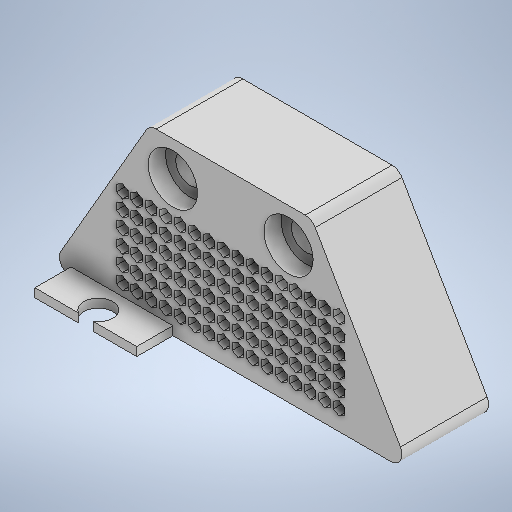
# Autodesk Inventor part: EngineMount
Saved by Autodesk Inventor 2026.1 (Build 301233020, 233B)
## iProperties
Created: 2025-10-14
Part Number: EngineMount
Material: Generic
Document SubType Name: Modeling
Designer: yo
Density: 1 g/cm^3
Appearance: Default
Author: yo
Autodesk Inventor part; units mm, degrees
ref_plane "YZ Plane" through (0, 0, 0) normal (1, 0, 0) x (0, 1, 0)
ref_plane "XZ Plane" through (0, 0, 0) normal (0, 1, 0) x (-1, 0, 0)
ref_plane "XY Plane" through (0, 0, 0) normal (0, 0, 1) x (1, 0, 0)
sketch "Sketch1" plane through (0, 0, 0) normal (0, 0, 1) x (1, 0, 0)
  line L0 (-55.2184, 0) -> (55.2184, 0)
  line L1 (-25.7735, 59) -> (25.7735, 59)
  circle A0 centre (-20, 47) radius 8.5
  line L2 (0, 59) -> (0, 0) construction
  circle A1 centre (-20, 47) radius 5
  circle A2 centre (20, 47) radius 8.5
  circle A3 centre (20, 47) radius 5
  arc A4 (-58.6825, 6) -> (-55.2184, 0) centre (-55.2184, 4) ccw
  arc A5 (-25.7735, 59) -> (-29.2376, 57) centre (-25.7735, 55) ccw
  line L3 (-58.6825, 6) -> (-29.2376, 57)
  arc A6 (55.2184, 0) -> (58.6825, 6) centre (55.2184, 4) ccw
  arc A7 (29.2376, 57) -> (25.7735, 59) centre (25.7735, 55) ccw
  line L4 (58.6825, 6) -> (29.2376, 57)
  line L5 (-55.2184, 3) -> (-20, 3)
  line L6 (-20, 3) -> (-20, 0)
  line L7 (-20, 0) -> (-55.2184, 0)
  line L8 (-55.2184, 0) -> (-55.2184, 3)
  line L9 (-35.5, 33.3453) -> (-37.5, 32.1906)
  line L10 (-37.5, 32.1906) -> (-39.5, 33.3453)
  line L11 (-39.5, 33.3453) -> (-39.5, 35.6547)
  line L12 (-39.5, 35.6547) -> (-37.5, 36.8094)
  line L13 (-37.5, 36.8094) -> (-35.5, 35.6547)
  line L14 (-35.5, 35.6547) -> (-35.5, 33.3453)
  line L15 (-32.5, 36.8094) -> (-30.5, 35.6547)
  line L16 (-34.5, 33.3453) -> (-34.5, 35.6547)
  line L17 (-30.5, 35.6547) -> (-30.5, 33.3453)
  line L18 (-32.5, 32.1906) -> (-34.5, 33.3453)
  line L19 (-30.5, 33.3453) -> (-32.5, 32.1906)
  line L20 (-34.5, 35.6547) -> (-32.5, 36.8094)
  line L21 (-27.5, 36.8094) -> (-25.5, 35.6547)
  line L22 (-29.5, 33.3453) -> (-29.5, 35.6547)
  line L23 (-25.5, 35.6547) -> (-25.5, 33.3453)
  line L24 (-27.5, 32.1906) -> (-29.5, 33.3453)
  line L25 (-25.5, 33.3453) -> (-27.5, 32.1906)
  line L26 (-29.5, 35.6547) -> (-27.5, 36.8094)
  line L27 (-22.5, 36.8094) -> (-20.5, 35.6547)
  line L28 (-24.5, 33.3453) -> (-24.5, 35.6547)
  line L29 (-20.5, 35.6547) -> (-20.5, 33.3453)
  line L30 (-22.5, 32.1906) -> (-24.5, 33.3453)
  line L31 (-20.5, 33.3453) -> (-22.5, 32.1906)
  line L32 (-24.5, 35.6547) -> (-22.5, 36.8094)
  line L33 (-17.5, 36.8094) -> (-15.5, 35.6547)
  line L34 (-19.5, 33.3453) -> (-19.5, 35.6547)
  line L35 (-15.5, 35.6547) -> (-15.5, 33.3453)
  line L36 (-17.5, 32.1906) -> (-19.5, 33.3453)
  line L37 (-15.5, 33.3453) -> (-17.5, 32.1906)
  line L38 (-19.5, 35.6547) -> (-17.5, 36.8094)
  line L39 (-12.5, 36.8094) -> (-10.5, 35.6547)
  line L40 (-14.5, 33.3453) -> (-14.5, 35.6547)
  line L41 (-10.5, 35.6547) -> (-10.5, 33.3453)
  line L42 (-12.5, 32.1906) -> (-14.5, 33.3453)
  line L43 (-10.5, 33.3453) -> (-12.5, 32.1906)
  line L44 (-14.5, 35.6547) -> (-12.5, 36.8094)
  line L45 (-7.5, 36.8094) -> (-5.5, 35.6547)
  line L46 (-9.5, 33.3453) -> (-9.5, 35.6547)
  line L47 (-5.5, 35.6547) -> (-5.5, 33.3453)
  line L48 (-7.5, 32.1906) -> (-9.5, 33.3453)
  line L49 (-5.5, 33.3453) -> (-7.5, 32.1906)
  line L50 (-9.5, 35.6547) -> (-7.5, 36.8094)
  line L51 (-2.5, 36.8094) -> (-0.5, 35.6547)
  line L52 (-4.5, 33.3453) -> (-4.5, 35.6547)
  line L53 (-0.5, 35.6547) -> (-0.5, 33.3453)
  line L54 (-2.5, 32.1906) -> (-4.5, 33.3453)
  line L55 (-0.5, 33.3453) -> (-2.5, 32.1906)
  line L56 (-4.5, 35.6547) -> (-2.5, 36.8094)
  line L57 (2.5, 36.8094) -> (4.5, 35.6547)
  line L58 (0.5, 33.3453) -> (0.5, 35.6547)
  line L59 (4.5, 35.6547) -> (4.5, 33.3453)
  line L60 (2.5, 32.1906) -> (0.5, 33.3453)
  line L61 (4.5, 33.3453) -> (2.5, 32.1906)
  line L62 (0.5, 35.6547) -> (2.5, 36.8094)
  line L63 (7.5, 36.8094) -> (9.5, 35.6547)
  line L64 (5.5, 33.3453) -> (5.5, 35.6547)
  line L65 (9.5, 35.6547) -> (9.5, 33.3453)
  line L66 (7.5, 32.1906) -> (5.5, 33.3453)
  line L67 (9.5, 33.3453) -> (7.5, 32.1906)
  line L68 (5.5, 35.6547) -> (7.5, 36.8094)
  line L69 (12.5, 36.8094) -> (14.5, 35.6547)
  line L70 (10.5, 33.3453) -> (10.5, 35.6547)
  line L71 (14.5, 35.6547) -> (14.5, 33.3453)
  line L72 (12.5, 32.1906) -> (10.5, 33.3453)
  line L73 (14.5, 33.3453) -> (12.5, 32.1906)
  line L74 (10.5, 35.6547) -> (12.5, 36.8094)
  line L75 (17.5, 36.8094) -> (19.5, 35.6547)
  line L76 (15.5, 33.3453) -> (15.5, 35.6547)
  line L77 (19.5, 35.6547) -> (19.5, 33.3453)
  line L78 (17.5, 32.1906) -> (15.5, 33.3453)
  line L79 (19.5, 33.3453) -> (17.5, 32.1906)
  line L80 (15.5, 35.6547) -> (17.5, 36.8094)
  line L81 (22.5, 36.8094) -> (24.5, 35.6547)
  line L82 (20.5, 33.3453) -> (20.5, 35.6547)
  line L83 (24.5, 35.6547) -> (24.5, 33.3453)
  line L84 (22.5, 32.1906) -> (20.5, 33.3453)
  line L85 (24.5, 33.3453) -> (22.5, 32.1906)
  line L86 (20.5, 35.6547) -> (22.5, 36.8094)
  line L87 (27.5, 36.8094) -> (29.5, 35.6547)
  line L88 (25.5, 33.3453) -> (25.5, 35.6547)
  line L89 (29.5, 35.6547) -> (29.5, 33.3453)
  line L90 (27.5, 32.1906) -> (25.5, 33.3453)
  line L91 (29.5, 33.3453) -> (27.5, 32.1906)
  line L92 (25.5, 35.6547) -> (27.5, 36.8094)
  line L93 (32.5, 36.8094) -> (34.5, 35.6547)
  line L94 (30.5, 33.3453) -> (30.5, 35.6547)
  line L95 (34.5, 35.6547) -> (34.5, 33.3453)
  line L96 (32.5, 32.1906) -> (30.5, 33.3453)
  line L97 (34.5, 33.3453) -> (32.5, 32.1906)
  line L98 (30.5, 35.6547) -> (32.5, 36.8094)
  line L99 (37.5, 36.8094) -> (39.5, 35.6547)
  line L100 (35.5, 33.3453) -> (35.5, 35.6547)
  line L101 (39.5, 35.6547) -> (39.5, 33.3453)
  line L102 (37.5, 32.1906) -> (35.5, 33.3453)
  line L103 (39.5, 33.3453) -> (37.5, 32.1906)
  line L104 (35.5, 35.6547) -> (37.5, 36.8094)
  line L105 (-37.5, 31.3094) -> (-35.5, 30.1547)
  line L106 (-39.5, 27.8453) -> (-39.5, 30.1547)
  line L107 (-35.5, 30.1547) -> (-35.5, 27.8453)
  line L108 (-37.5, 26.6906) -> (-39.5, 27.8453)
  line L109 (-35.5, 27.8453) -> (-37.5, 26.6906)
  line L110 (-39.5, 30.1547) -> (-37.5, 31.3094)
  line L111 (-32.5, 31.3094) -> (-30.5, 30.1547)
  line L112 (-34.5, 27.8453) -> (-34.5, 30.1547)
  line L113 (-30.5, 30.1547) -> (-30.5, 27.8453)
  line L114 (-32.5, 26.6906) -> (-34.5, 27.8453)
  line L115 (-30.5, 27.8453) -> (-32.5, 26.6906)
  line L116 (-34.5, 30.1547) -> (-32.5, 31.3094)
  line L117 (-27.5, 31.3094) -> (-25.5, 30.1547)
  line L118 (-29.5, 27.8453) -> (-29.5, 30.1547)
  line L119 (-25.5, 30.1547) -> (-25.5, 27.8453)
  line L120 (-27.5, 26.6906) -> (-29.5, 27.8453)
  line L121 (-25.5, 27.8453) -> (-27.5, 26.6906)
  line L122 (-29.5, 30.1547) -> (-27.5, 31.3094)
  line L123 (-22.5, 31.3094) -> (-20.5, 30.1547)
  line L124 (-24.5, 27.8453) -> (-24.5, 30.1547)
  line L125 (-20.5, 30.1547) -> (-20.5, 27.8453)
  line L126 (-22.5, 26.6906) -> (-24.5, 27.8453)
  line L127 (-20.5, 27.8453) -> (-22.5, 26.6906)
  line L128 (-24.5, 30.1547) -> (-22.5, 31.3094)
  line L129 (-17.5, 31.3094) -> (-15.5, 30.1547)
  line L130 (-19.5, 27.8453) -> (-19.5, 30.1547)
  line L131 (-15.5, 30.1547) -> (-15.5, 27.8453)
  line L132 (-17.5, 26.6906) -> (-19.5, 27.8453)
  line L133 (-15.5, 27.8453) -> (-17.5, 26.6906)
  line L134 (-19.5, 30.1547) -> (-17.5, 31.3094)
  line L135 (-12.5, 31.3094) -> (-10.5, 30.1547)
  line L136 (-14.5, 27.8453) -> (-14.5, 30.1547)
  line L137 (-10.5, 30.1547) -> (-10.5, 27.8453)
  line L138 (-12.5, 26.6906) -> (-14.5, 27.8453)
  line L139 (-10.5, 27.8453) -> (-12.5, 26.6906)
  line L140 (-14.5, 30.1547) -> (-12.5, 31.3094)
  line L141 (-7.5, 31.3094) -> (-5.5, 30.1547)
  line L142 (-9.5, 27.8453) -> (-9.5, 30.1547)
  line L143 (-5.5, 30.1547) -> (-5.5, 27.8453)
  line L144 (-7.5, 26.6906) -> (-9.5, 27.8453)
  line L145 (-5.5, 27.8453) -> (-7.5, 26.6906)
  line L146 (-9.5, 30.1547) -> (-7.5, 31.3094)
  line L147 (-2.5, 31.3094) -> (-0.5, 30.1547)
  line L148 (-4.5, 27.8453) -> (-4.5, 30.1547)
  line L149 (-0.5, 30.1547) -> (-0.5, 27.8453)
  line L150 (-2.5, 26.6906) -> (-4.5, 27.8453)
  line L151 (-0.5, 27.8453) -> (-2.5, 26.6906)
  line L152 (-4.5, 30.1547) -> (-2.5, 31.3094)
  line L153 (2.5, 31.3094) -> (4.5, 30.1547)
  line L154 (0.5, 27.8453) -> (0.5, 30.1547)
  line L155 (4.5, 30.1547) -> (4.5, 27.8453)
  line L156 (2.5, 26.6906) -> (0.5, 27.8453)
  line L157 (4.5, 27.8453) -> (2.5, 26.6906)
  line L158 (0.5, 30.1547) -> (2.5, 31.3094)
  line L159 (7.5, 31.3094) -> (9.5, 30.1547)
  line L160 (5.5, 27.8453) -> (5.5, 30.1547)
  line L161 (9.5, 30.1547) -> (9.5, 27.8453)
  line L162 (7.5, 26.6906) -> (5.5, 27.8453)
  line L163 (9.5, 27.8453) -> (7.5, 26.6906)
  line L164 (5.5, 30.1547) -> (7.5, 31.3094)
  line L165 (12.5, 31.3094) -> (14.5, 30.1547)
  line L166 (10.5, 27.8453) -> (10.5, 30.1547)
  line L167 (14.5, 30.1547) -> (14.5, 27.8453)
  line L168 (12.5, 26.6906) -> (10.5, 27.8453)
  line L169 (14.5, 27.8453) -> (12.5, 26.6906)
  line L170 (10.5, 30.1547) -> (12.5, 31.3094)
  line L171 (17.5, 31.3094) -> (19.5, 30.1547)
  line L172 (15.5, 27.8453) -> (15.5, 30.1547)
  line L173 (19.5, 30.1547) -> (19.5, 27.8453)
  line L174 (17.5, 26.6906) -> (15.5, 27.8453)
  line L175 (19.5, 27.8453) -> (17.5, 26.6906)
  line L176 (15.5, 30.1547) -> (17.5, 31.3094)
  line L177 (22.5, 31.3094) -> (24.5, 30.1547)
  line L178 (20.5, 27.8453) -> (20.5, 30.1547)
  line L179 (24.5, 30.1547) -> (24.5, 27.8453)
  line L180 (22.5, 26.6906) -> (20.5, 27.8453)
  line L181 (24.5, 27.8453) -> (22.5, 26.6906)
  line L182 (20.5, 30.1547) -> (22.5, 31.3094)
  line L183 (27.5, 31.3094) -> (29.5, 30.1547)
  line L184 (25.5, 27.8453) -> (25.5, 30.1547)
  line L185 (29.5, 30.1547) -> (29.5, 27.8453)
  line L186 (27.5, 26.6906) -> (25.5, 27.8453)
  line L187 (29.5, 27.8453) -> (27.5, 26.6906)
  line L188 (25.5, 30.1547) -> (27.5, 31.3094)
  line L189 (32.5, 31.3094) -> (34.5, 30.1547)
  line L190 (30.5, 27.8453) -> (30.5, 30.1547)
  line L191 (34.5, 30.1547) -> (34.5, 27.8453)
  line L192 (32.5, 26.6906) -> (30.5, 27.8453)
  line L193 (34.5, 27.8453) -> (32.5, 26.6906)
  line L194 (30.5, 30.1547) -> (32.5, 31.3094)
  line L195 (37.5, 31.3094) -> (39.5, 30.1547)
  line L196 (35.5, 27.8453) -> (35.5, 30.1547)
  line L197 (39.5, 30.1547) -> (39.5, 27.8453)
  line L198 (37.5, 26.6906) -> (35.5, 27.8453)
  line L199 (39.5, 27.8453) -> (37.5, 26.6906)
  line L200 (35.5, 30.1547) -> (37.5, 31.3094)
  line L201 (-37.5, 25.8094) -> (-35.5, 24.6547)
  line L202 (-39.5, 22.3453) -> (-39.5, 24.6547)
  line L203 (-35.5, 24.6547) -> (-35.5, 22.3453)
  line L204 (-37.5, 21.1906) -> (-39.5, 22.3453)
  line L205 (-35.5, 22.3453) -> (-37.5, 21.1906)
  line L206 (-39.5, 24.6547) -> (-37.5, 25.8094)
  line L207 (-32.5, 25.8094) -> (-30.5, 24.6547)
  line L208 (-34.5, 22.3453) -> (-34.5, 24.6547)
  line L209 (-30.5, 24.6547) -> (-30.5, 22.3453)
  line L210 (-32.5, 21.1906) -> (-34.5, 22.3453)
  line L211 (-30.5, 22.3453) -> (-32.5, 21.1906)
  line L212 (-34.5, 24.6547) -> (-32.5, 25.8094)
  line L213 (-27.5, 25.8094) -> (-25.5, 24.6547)
  line L214 (-29.5, 22.3453) -> (-29.5, 24.6547)
  line L215 (-25.5, 24.6547) -> (-25.5, 22.3453)
  line L216 (-27.5, 21.1906) -> (-29.5, 22.3453)
  line L217 (-25.5, 22.3453) -> (-27.5, 21.1906)
  line L218 (-29.5, 24.6547) -> (-27.5, 25.8094)
  line L219 (-22.5, 25.8094) -> (-20.5, 24.6547)
  line L220 (-24.5, 22.3453) -> (-24.5, 24.6547)
  line L221 (-20.5, 24.6547) -> (-20.5, 22.3453)
  line L222 (-22.5, 21.1906) -> (-24.5, 22.3453)
  line L223 (-20.5, 22.3453) -> (-22.5, 21.1906)
  line L224 (-24.5, 24.6547) -> (-22.5, 25.8094)
  line L225 (-17.5, 25.8094) -> (-15.5, 24.6547)
  line L226 (-19.5, 22.3453) -> (-19.5, 24.6547)
  line L227 (-15.5, 24.6547) -> (-15.5, 22.3453)
  line L228 (-17.5, 21.1906) -> (-19.5, 22.3453)
  line L229 (-15.5, 22.3453) -> (-17.5, 21.1906)
  line L230 (-19.5, 24.6547) -> (-17.5, 25.8094)
  line L231 (-12.5, 25.8094) -> (-10.5, 24.6547)
  line L232 (-14.5, 22.3453) -> (-14.5, 24.6547)
  line L233 (-10.5, 24.6547) -> (-10.5, 22.3453)
  line L234 (-12.5, 21.1906) -> (-14.5, 22.3453)
  line L235 (-10.5, 22.3453) -> (-12.5, 21.1906)
  line L236 (-14.5, 24.6547) -> (-12.5, 25.8094)
  line L237 (-7.5, 25.8094) -> (-5.5, 24.6547)
  line L238 (-9.5, 22.3453) -> (-9.5, 24.6547)
  line L239 (-5.5, 24.6547) -> (-5.5, 22.3453)
  line L240 (-7.5, 21.1906) -> (-9.5, 22.3453)
  line L241 (-5.5, 22.3453) -> (-7.5, 21.1906)
  line L242 (-9.5, 24.6547) -> (-7.5, 25.8094)
  line L243 (-2.5, 25.8094) -> (-0.5, 24.6547)
  line L244 (-4.5, 22.3453) -> (-4.5, 24.6547)
  line L245 (-0.5, 24.6547) -> (-0.5, 22.3453)
  line L246 (-2.5, 21.1906) -> (-4.5, 22.3453)
  line L247 (-0.5, 22.3453) -> (-2.5, 21.1906)
  line L248 (-4.5, 24.6547) -> (-2.5, 25.8094)
  line L249 (2.5, 25.8094) -> (4.5, 24.6547)
  line L250 (0.5, 22.3453) -> (0.5, 24.6547)
  line L251 (4.5, 24.6547) -> (4.5, 22.3453)
  line L252 (2.5, 21.1906) -> (0.5, 22.3453)
  line L253 (4.5, 22.3453) -> (2.5, 21.1906)
  line L254 (0.5, 24.6547) -> (2.5, 25.8094)
  line L255 (7.5, 25.8094) -> (9.5, 24.6547)
  line L256 (5.5, 22.3453) -> (5.5, 24.6547)
  line L257 (9.5, 24.6547) -> (9.5, 22.3453)
  line L258 (7.5, 21.1906) -> (5.5, 22.3453)
  line L259 (9.5, 22.3453) -> (7.5, 21.1906)
  line L260 (5.5, 24.6547) -> (7.5, 25.8094)
  line L261 (12.5, 25.8094) -> (14.5, 24.6547)
  line L262 (10.5, 22.3453) -> (10.5, 24.6547)
  line L263 (14.5, 24.6547) -> (14.5, 22.3453)
  line L264 (12.5, 21.1906) -> (10.5, 22.3453)
  line L265 (14.5, 22.3453) -> (12.5, 21.1906)
  line L266 (10.5, 24.6547) -> (12.5, 25.8094)
  line L267 (17.5, 25.8094) -> (19.5, 24.6547)
  line L268 (15.5, 22.3453) -> (15.5, 24.6547)
  line L269 (19.5, 24.6547) -> (19.5, 22.3453)
  line L270 (17.5, 21.1906) -> (15.5, 22.3453)
  line L271 (19.5, 22.3453) -> (17.5, 21.1906)
  line L272 (15.5, 24.6547) -> (17.5, 25.8094)
  line L273 (22.5, 25.8094) -> (24.5, 24.6547)
  line L274 (20.5, 22.3453) -> (20.5, 24.6547)
  line L275 (24.5, 24.6547) -> (24.5, 22.3453)
  line L276 (22.5, 21.1906) -> (20.5, 22.3453)
  line L277 (24.5, 22.3453) -> (22.5, 21.1906)
  line L278 (20.5, 24.6547) -> (22.5, 25.8094)
  line L279 (27.5, 25.8094) -> (29.5, 24.6547)
  line L280 (25.5, 22.3453) -> (25.5, 24.6547)
  line L281 (29.5, 24.6547) -> (29.5, 22.3453)
  line L282 (27.5, 21.1906) -> (25.5, 22.3453)
  line L283 (29.5, 22.3453) -> (27.5, 21.1906)
  line L284 (25.5, 24.6547) -> (27.5, 25.8094)
  line L285 (32.5, 25.8094) -> (34.5, 24.6547)
  line L286 (30.5, 22.3453) -> (30.5, 24.6547)
  line L287 (34.5, 24.6547) -> (34.5, 22.3453)
  line L288 (32.5, 21.1906) -> (30.5, 22.3453)
  line L289 (34.5, 22.3453) -> (32.5, 21.1906)
  line L290 (30.5, 24.6547) -> (32.5, 25.8094)
  line L291 (37.5, 25.8094) -> (39.5, 24.6547)
  line L292 (35.5, 22.3453) -> (35.5, 24.6547)
  line L293 (39.5, 24.6547) -> (39.5, 22.3453)
  line L294 (37.5, 21.1906) -> (35.5, 22.3453)
  line L295 (39.5, 22.3453) -> (37.5, 21.1906)
  line L296 (35.5, 24.6547) -> (37.5, 25.8094)
  line L297 (-37.5, 20.3094) -> (-35.5, 19.1547)
  line L298 (-39.5, 16.8453) -> (-39.5, 19.1547)
  line L299 (-35.5, 19.1547) -> (-35.5, 16.8453)
  line L300 (-37.5, 15.6906) -> (-39.5, 16.8453)
  line L301 (-35.5, 16.8453) -> (-37.5, 15.6906)
  line L302 (-39.5, 19.1547) -> (-37.5, 20.3094)
  line L303 (-32.5, 20.3094) -> (-30.5, 19.1547)
  line L304 (-34.5, 16.8453) -> (-34.5, 19.1547)
  line L305 (-30.5, 19.1547) -> (-30.5, 16.8453)
  line L306 (-32.5, 15.6906) -> (-34.5, 16.8453)
  line L307 (-30.5, 16.8453) -> (-32.5, 15.6906)
  line L308 (-34.5, 19.1547) -> (-32.5, 20.3094)
  line L309 (-27.5, 20.3094) -> (-25.5, 19.1547)
  line L310 (-29.5, 16.8453) -> (-29.5, 19.1547)
  line L311 (-25.5, 19.1547) -> (-25.5, 16.8453)
  line L312 (-27.5, 15.6906) -> (-29.5, 16.8453)
  line L313 (-25.5, 16.8453) -> (-27.5, 15.6906)
  line L314 (-29.5, 19.1547) -> (-27.5, 20.3094)
  line L315 (-22.5, 20.3094) -> (-20.5, 19.1547)
  line L316 (-24.5, 16.8453) -> (-24.5, 19.1547)
  line L317 (-20.5, 19.1547) -> (-20.5, 16.8453)
  line L318 (-22.5, 15.6906) -> (-24.5, 16.8453)
  line L319 (-20.5, 16.8453) -> (-22.5, 15.6906)
  line L320 (-24.5, 19.1547) -> (-22.5, 20.3094)
  line L321 (-17.5, 20.3094) -> (-15.5, 19.1547)
  line L322 (-19.5, 16.8453) -> (-19.5, 19.1547)
  line L323 (-15.5, 19.1547) -> (-15.5, 16.8453)
  line L324 (-17.5, 15.6906) -> (-19.5, 16.8453)
  line L325 (-15.5, 16.8453) -> (-17.5, 15.6906)
  line L326 (-19.5, 19.1547) -> (-17.5, 20.3094)
  line L327 (-12.5, 20.3094) -> (-10.5, 19.1547)
  line L328 (-14.5, 16.8453) -> (-14.5, 19.1547)
  line L329 (-10.5, 19.1547) -> (-10.5, 16.8453)
  line L330 (-12.5, 15.6906) -> (-14.5, 16.8453)
  line L331 (-10.5, 16.8453) -> (-12.5, 15.6906)
  line L332 (-14.5, 19.1547) -> (-12.5, 20.3094)
  line L333 (-7.5, 20.3094) -> (-5.5, 19.1547)
  line L334 (-9.5, 16.8453) -> (-9.5, 19.1547)
  line L335 (-5.5, 19.1547) -> (-5.5, 16.8453)
  line L336 (-7.5, 15.6906) -> (-9.5, 16.8453)
  line L337 (-5.5, 16.8453) -> (-7.5, 15.6906)
  line L338 (-9.5, 19.1547) -> (-7.5, 20.3094)
  line L339 (-2.5, 20.3094) -> (-0.5, 19.1547)
  line L340 (-4.5, 16.8453) -> (-4.5, 19.1547)
  line L341 (-0.5, 19.1547) -> (-0.5, 16.8453)
  line L342 (-2.5, 15.6906) -> (-4.5, 16.8453)
  line L343 (-0.5, 16.8453) -> (-2.5, 15.6906)
  line L344 (-4.5, 19.1547) -> (-2.5, 20.3094)
  line L345 (2.5, 20.3094) -> (4.5, 19.1547)
  line L346 (0.5, 16.8453) -> (0.5, 19.1547)
  line L347 (4.5, 19.1547) -> (4.5, 16.8453)
  line L348 (2.5, 15.6906) -> (0.5, 16.8453)
  line L349 (4.5, 16.8453) -> (2.5, 15.6906)
  line L350 (0.5, 19.1547) -> (2.5, 20.3094)
  line L351 (7.5, 20.3094) -> (9.5, 19.1547)
  line L352 (5.5, 16.8453) -> (5.5, 19.1547)
  line L353 (9.5, 19.1547) -> (9.5, 16.8453)
  line L354 (7.5, 15.6906) -> (5.5, 16.8453)
  line L355 (9.5, 16.8453) -> (7.5, 15.6906)
  line L356 (5.5, 19.1547) -> (7.5, 20.3094)
  line L357 (12.5, 20.3094) -> (14.5, 19.1547)
  line L358 (10.5, 16.8453) -> (10.5, 19.1547)
  line L359 (14.5, 19.1547) -> (14.5, 16.8453)
  line L360 (12.5, 15.6906) -> (10.5, 16.8453)
  line L361 (14.5, 16.8453) -> (12.5, 15.6906)
  line L362 (10.5, 19.1547) -> (12.5, 20.3094)
  line L363 (17.5, 20.3094) -> (19.5, 19.1547)
  line L364 (15.5, 16.8453) -> (15.5, 19.1547)
  line L365 (19.5, 19.1547) -> (19.5, 16.8453)
  line L366 (17.5, 15.6906) -> (15.5, 16.8453)
  line L367 (19.5, 16.8453) -> (17.5, 15.6906)
  line L368 (15.5, 19.1547) -> (17.5, 20.3094)
  line L369 (22.5, 20.3094) -> (24.5, 19.1547)
  line L370 (20.5, 16.8453) -> (20.5, 19.1547)
  line L371 (24.5, 19.1547) -> (24.5, 16.8453)
  line L372 (22.5, 15.6906) -> (20.5, 16.8453)
  line L373 (24.5, 16.8453) -> (22.5, 15.6906)
  line L374 (20.5, 19.1547) -> (22.5, 20.3094)
  line L375 (27.5, 20.3094) -> (29.5, 19.1547)
  line L376 (25.5, 16.8453) -> (25.5, 19.1547)
  line L377 (29.5, 19.1547) -> (29.5, 16.8453)
  line L378 (27.5, 15.6906) -> (25.5, 16.8453)
  line L379 (29.5, 16.8453) -> (27.5, 15.6906)
  line L380 (25.5, 19.1547) -> (27.5, 20.3094)
  line L381 (32.5, 20.3094) -> (34.5, 19.1547)
  line L382 (30.5, 16.8453) -> (30.5, 19.1547)
  line L383 (34.5, 19.1547) -> (34.5, 16.8453)
  line L384 (32.5, 15.6906) -> (30.5, 16.8453)
  line L385 (34.5, 16.8453) -> (32.5, 15.6906)
  line L386 (30.5, 19.1547) -> (32.5, 20.3094)
  line L387 (37.5, 20.3094) -> (39.5, 19.1547)
  line L388 (35.5, 16.8453) -> (35.5, 19.1547)
  line L389 (39.5, 19.1547) -> (39.5, 16.8453)
  line L390 (37.5, 15.6906) -> (35.5, 16.8453)
  line L391 (39.5, 16.8453) -> (37.5, 15.6906)
  line L392 (35.5, 19.1547) -> (37.5, 20.3094)
  line L393 (-20, 38.5) -> (0, 38.5) construction
  line L394 (-20, 3) -> (0, 3) construction
  line L395 (0, 38.5) -> (0, 3) construction
  line L396 (-37.5, 14.8094) -> (-35.5, 13.6547)
  line L397 (-39.5, 11.3453) -> (-39.5, 13.6547)
  line L398 (-35.5, 13.6547) -> (-35.5, 11.3453)
  line L399 (-37.5, 10.1906) -> (-39.5, 11.3453)
  line L400 (-35.5, 11.3453) -> (-37.5, 10.1906)
  line L401 (-39.5, 13.6547) -> (-37.5, 14.8094)
  line L402 (-32.5, 14.8094) -> (-30.5, 13.6547)
  line L403 (-34.5, 11.3453) -> (-34.5, 13.6547)
  line L404 (-30.5, 13.6547) -> (-30.5, 11.3453)
  line L405 (-32.5, 10.1906) -> (-34.5, 11.3453)
  line L406 (-30.5, 11.3453) -> (-32.5, 10.1906)
  line L407 (-34.5, 13.6547) -> (-32.5, 14.8094)
  line L408 (-27.5, 14.8094) -> (-25.5, 13.6547)
  line L409 (-29.5, 11.3453) -> (-29.5, 13.6547)
  line L410 (-25.5, 13.6547) -> (-25.5, 11.3453)
  line L411 (-27.5, 10.1906) -> (-29.5, 11.3453)
  line L412 (-25.5, 11.3453) -> (-27.5, 10.1906)
  line L413 (-29.5, 13.6547) -> (-27.5, 14.8094)
  line L414 (-22.5, 14.8094) -> (-20.5, 13.6547)
  line L415 (-24.5, 11.3453) -> (-24.5, 13.6547)
  line L416 (-20.5, 13.6547) -> (-20.5, 11.3453)
  line L417 (-22.5, 10.1906) -> (-24.5, 11.3453)
  line L418 (-20.5, 11.3453) -> (-22.5, 10.1906)
  line L419 (-24.5, 13.6547) -> (-22.5, 14.8094)
  line L420 (-17.5, 14.8094) -> (-15.5, 13.6547)
  line L421 (-19.5, 11.3453) -> (-19.5, 13.6547)
  line L422 (-15.5, 13.6547) -> (-15.5, 11.3453)
  line L423 (-17.5, 10.1906) -> (-19.5, 11.3453)
  line L424 (-15.5, 11.3453) -> (-17.5, 10.1906)
  line L425 (-19.5, 13.6547) -> (-17.5, 14.8094)
  line L426 (-12.5, 14.8094) -> (-10.5, 13.6547)
  line L427 (-14.5, 11.3453) -> (-14.5, 13.6547)
  line L428 (-10.5, 13.6547) -> (-10.5, 11.3453)
  line L429 (-12.5, 10.1906) -> (-14.5, 11.3453)
  line L430 (-10.5, 11.3453) -> (-12.5, 10.1906)
  line L431 (-14.5, 13.6547) -> (-12.5, 14.8094)
  line L432 (-7.5, 14.8094) -> (-5.5, 13.6547)
  line L433 (-9.5, 11.3453) -> (-9.5, 13.6547)
  line L434 (-5.5, 13.6547) -> (-5.5, 11.3453)
  line L435 (-7.5, 10.1906) -> (-9.5, 11.3453)
  line L436 (-5.5, 11.3453) -> (-7.5, 10.1906)
  line L437 (-9.5, 13.6547) -> (-7.5, 14.8094)
  line L438 (-2.5, 14.8094) -> (-0.5, 13.6547)
  line L439 (-4.5, 11.3453) -> (-4.5, 13.6547)
  line L440 (-0.5, 13.6547) -> (-0.5, 11.3453)
  line L441 (-2.5, 10.1906) -> (-4.5, 11.3453)
  line L442 (-0.5, 11.3453) -> (-2.5, 10.1906)
  line L443 (-4.5, 13.6547) -> (-2.5, 14.8094)
  line L444 (2.5, 14.8094) -> (4.5, 13.6547)
  line L445 (0.5, 11.3453) -> (0.5, 13.6547)
  line L446 (4.5, 13.6547) -> (4.5, 11.3453)
  line L447 (2.5, 10.1906) -> (0.5, 11.3453)
  line L448 (4.5, 11.3453) -> (2.5, 10.1906)
  line L449 (0.5, 13.6547) -> (2.5, 14.8094)
  line L450 (7.5, 14.8094) -> (9.5, 13.6547)
  line L451 (5.5, 11.3453) -> (5.5, 13.6547)
  line L452 (9.5, 13.6547) -> (9.5, 11.3453)
  line L453 (7.5, 10.1906) -> (5.5, 11.3453)
  line L454 (9.5, 11.3453) -> (7.5, 10.1906)
  line L455 (5.5, 13.6547) -> (7.5, 14.8094)
  line L456 (12.5, 14.8094) -> (14.5, 13.6547)
  line L457 (10.5, 11.3453) -> (10.5, 13.6547)
  line L458 (14.5, 13.6547) -> (14.5, 11.3453)
  line L459 (12.5, 10.1906) -> (10.5, 11.3453)
  line L460 (14.5, 11.3453) -> (12.5, 10.1906)
  line L461 (10.5, 13.6547) -> (12.5, 14.8094)
  line L462 (17.5, 14.8094) -> (19.5, 13.6547)
  line L463 (15.5, 11.3453) -> (15.5, 13.6547)
  line L464 (19.5, 13.6547) -> (19.5, 11.3453)
  line L465 (17.5, 10.1906) -> (15.5, 11.3453)
  line L466 (19.5, 11.3453) -> (17.5, 10.1906)
  line L467 (15.5, 13.6547) -> (17.5, 14.8094)
  line L468 (22.5, 14.8094) -> (24.5, 13.6547)
  line L469 (20.5, 11.3453) -> (20.5, 13.6547)
  line L470 (24.5, 13.6547) -> (24.5, 11.3453)
  line L471 (22.5, 10.1906) -> (20.5, 11.3453)
  line L472 (24.5, 11.3453) -> (22.5, 10.1906)
  line L473 (20.5, 13.6547) -> (22.5, 14.8094)
  line L474 (27.5, 14.8094) -> (29.5, 13.6547)
  line L475 (25.5, 11.3453) -> (25.5, 13.6547)
  line L476 (29.5, 13.6547) -> (29.5, 11.3453)
  line L477 (27.5, 10.1906) -> (25.5, 11.3453)
  line L478 (29.5, 11.3453) -> (27.5, 10.1906)
  line L479 (25.5, 13.6547) -> (27.5, 14.8094)
  line L480 (32.5, 14.8094) -> (34.5, 13.6547)
  line L481 (30.5, 11.3453) -> (30.5, 13.6547)
  line L482 (34.5, 13.6547) -> (34.5, 11.3453)
  line L483 (32.5, 10.1906) -> (30.5, 11.3453)
  line L484 (34.5, 11.3453) -> (32.5, 10.1906)
  line L485 (30.5, 13.6547) -> (32.5, 14.8094)
  line L486 (37.5, 14.8094) -> (39.5, 13.6547)
  line L487 (35.5, 11.3453) -> (35.5, 13.6547)
  line L488 (39.5, 13.6547) -> (39.5, 11.3453)
  line L489 (37.5, 10.1906) -> (35.5, 11.3453)
  line L490 (39.5, 11.3453) -> (37.5, 10.1906)
  line L491 (35.5, 13.6547) -> (37.5, 14.8094)
  line L492 (-37.5, 9.3094) -> (-35.5, 8.1547)
  line L493 (-39.5, 5.8453) -> (-39.5, 8.1547)
  line L494 (-35.5, 8.1547) -> (-35.5, 5.8453)
  line L495 (-37.5, 4.6906) -> (-39.5, 5.8453)
  line L496 (-35.5, 5.8453) -> (-37.5, 4.6906)
  line L497 (-39.5, 8.1547) -> (-37.5, 9.3094)
  line L498 (-32.5, 9.3094) -> (-30.5, 8.1547)
  line L499 (-34.5, 5.8453) -> (-34.5, 8.1547)
  line L500 (-30.5, 8.1547) -> (-30.5, 5.8453)
  line L501 (-32.5, 4.6906) -> (-34.5, 5.8453)
  line L502 (-30.5, 5.8453) -> (-32.5, 4.6906)
  line L503 (-34.5, 8.1547) -> (-32.5, 9.3094)
  line L504 (-27.5, 9.3094) -> (-25.5, 8.1547)
  line L505 (-29.5, 5.8453) -> (-29.5, 8.1547)
  line L506 (-25.5, 8.1547) -> (-25.5, 5.8453)
  line L507 (-27.5, 4.6906) -> (-29.5, 5.8453)
  line L508 (-25.5, 5.8453) -> (-27.5, 4.6906)
  line L509 (-29.5, 8.1547) -> (-27.5, 9.3094)
  line L510 (-22.5, 9.3094) -> (-20.5, 8.1547)
  line L511 (-24.5, 5.8453) -> (-24.5, 8.1547)
  line L512 (-20.5, 8.1547) -> (-20.5, 5.8453)
  line L513 (-22.5, 4.6906) -> (-24.5, 5.8453)
  line L514 (-20.5, 5.8453) -> (-22.5, 4.6906)
  line L515 (-24.5, 8.1547) -> (-22.5, 9.3094)
  line L516 (-17.5, 9.3094) -> (-15.5, 8.1547)
  line L517 (-19.5, 5.8453) -> (-19.5, 8.1547)
  line L518 (-15.5, 8.1547) -> (-15.5, 5.8453)
  line L519 (-17.5, 4.6906) -> (-19.5, 5.8453)
  line L520 (-15.5, 5.8453) -> (-17.5, 4.6906)
  line L521 (-19.5, 8.1547) -> (-17.5, 9.3094)
  line L522 (-12.5, 9.3094) -> (-10.5, 8.1547)
  line L523 (-14.5, 5.8453) -> (-14.5, 8.1547)
  line L524 (-10.5, 8.1547) -> (-10.5, 5.8453)
  line L525 (-12.5, 4.6906) -> (-14.5, 5.8453)
  line L526 (-10.5, 5.8453) -> (-12.5, 4.6906)
  line L527 (-14.5, 8.1547) -> (-12.5, 9.3094)
  line L528 (-7.5, 9.3094) -> (-5.5, 8.1547)
  line L529 (-9.5, 5.8453) -> (-9.5, 8.1547)
  line L530 (-5.5, 8.1547) -> (-5.5, 5.8453)
  line L531 (-7.5, 4.6906) -> (-9.5, 5.8453)
  line L532 (-5.5, 5.8453) -> (-7.5, 4.6906)
  line L533 (-9.5, 8.1547) -> (-7.5, 9.3094)
  line L534 (-2.5, 9.3094) -> (-0.5, 8.1547)
  line L535 (-4.5, 5.8453) -> (-4.5, 8.1547)
  line L536 (-0.5, 8.1547) -> (-0.5, 5.8453)
  line L537 (-2.5, 4.6906) -> (-4.5, 5.8453)
  line L538 (-0.5, 5.8453) -> (-2.5, 4.6906)
  line L539 (-4.5, 8.1547) -> (-2.5, 9.3094)
  line L540 (2.5, 9.3094) -> (4.5, 8.1547)
  line L541 (0.5, 5.8453) -> (0.5, 8.1547)
  line L542 (4.5, 8.1547) -> (4.5, 5.8453)
  line L543 (2.5, 4.6906) -> (0.5, 5.8453)
  line L544 (4.5, 5.8453) -> (2.5, 4.6906)
  line L545 (0.5, 8.1547) -> (2.5, 9.3094)
  line L546 (7.5, 9.3094) -> (9.5, 8.1547)
  line L547 (5.5, 5.8453) -> (5.5, 8.1547)
  line L548 (9.5, 8.1547) -> (9.5, 5.8453)
  line L549 (7.5, 4.6906) -> (5.5, 5.8453)
  line L550 (9.5, 5.8453) -> (7.5, 4.6906)
  line L551 (5.5, 8.1547) -> (7.5, 9.3094)
  line L552 (12.5, 9.3094) -> (14.5, 8.1547)
  line L553 (10.5, 5.8453) -> (10.5, 8.1547)
  line L554 (14.5, 8.1547) -> (14.5, 5.8453)
  line L555 (12.5, 4.6906) -> (10.5, 5.8453)
  line L556 (14.5, 5.8453) -> (12.5, 4.6906)
  line L557 (10.5, 8.1547) -> (12.5, 9.3094)
  line L558 (17.5, 9.3094) -> (19.5, 8.1547)
  line L559 (15.5, 5.8453) -> (15.5, 8.1547)
  line L560 (19.5, 8.1547) -> (19.5, 5.8453)
  line L561 (17.5, 4.6906) -> (15.5, 5.8453)
  line L562 (19.5, 5.8453) -> (17.5, 4.6906)
  line L563 (15.5, 8.1547) -> (17.5, 9.3094)
  line L564 (22.5, 9.3094) -> (24.5, 8.1547)
  line L565 (20.5, 5.8453) -> (20.5, 8.1547)
  line L566 (24.5, 8.1547) -> (24.5, 5.8453)
  line L567 (22.5, 4.6906) -> (20.5, 5.8453)
  line L568 (24.5, 5.8453) -> (22.5, 4.6906)
  line L569 (20.5, 8.1547) -> (22.5, 9.3094)
  line L570 (27.5, 9.3094) -> (29.5, 8.1547)
  line L571 (25.5, 5.8453) -> (25.5, 8.1547)
  line L572 (29.5, 8.1547) -> (29.5, 5.8453)
  line L573 (27.5, 4.6906) -> (25.5, 5.8453)
  line L574 (29.5, 5.8453) -> (27.5, 4.6906)
  line L575 (25.5, 8.1547) -> (27.5, 9.3094)
  line L576 (32.5, 9.3094) -> (34.5, 8.1547)
  line L577 (30.5, 5.8453) -> (30.5, 8.1547)
  line L578 (34.5, 8.1547) -> (34.5, 5.8453)
  line L579 (32.5, 4.6906) -> (30.5, 5.8453)
  line L580 (34.5, 5.8453) -> (32.5, 4.6906)
  line L581 (30.5, 8.1547) -> (32.5, 9.3094)
  line L582 (37.5, 9.3094) -> (39.5, 8.1547)
  line L583 (35.5, 5.8453) -> (35.5, 8.1547)
  line L584 (39.5, 8.1547) -> (39.5, 5.8453)
  line L585 (37.5, 4.6906) -> (35.5, 5.8453)
  line L586 (39.5, 5.8453) -> (37.5, 4.6906)
  line L587 (35.5, 8.1547) -> (37.5, 9.3094)
  line L588 (39.5, 4.6906) -> (-39.5, 4.6906) construction
  line L589 (-39.5, 4.6906) -> (-39.5, 36.8094) construction
  line L590 (-39.5, 36.8094) -> (39.5, 36.8094) construction
  line L591 (39.5, 36.8094) -> (39.5, 4.6906) construction
  point P0 (-55.2184, 1.5)
  point P1 (-37.6092, 0)
  point P2 (-20, 0)
  point P3 (-20, 1.5)
  point P4 (-37.5, 34.5)
  point P5 (-32.5, 34.5)
  point P6 (-27.5, 34.5)
  point P7 (-22.5, 34.5)
  point P8 (-17.5, 34.5)
  point P9 (-12.5, 34.5)
  point P10 (-7.5, 34.5)
  point P11 (-2.5, 34.5)
  point P12 (2.5, 34.5)
  point P13 (7.5, 34.5)
  point P14 (12.5, 34.5)
  point P15 (17.5, 34.5)
  point P16 (22.5, 34.5)
  point P17 (27.5, 34.5)
  point P18 (32.5, 34.5)
  point P19 (37.5, 34.5)
  point P20 (-37.5, 29)
  point P21 (-32.5, 29)
  point P22 (-27.5, 29)
  point P23 (-22.5, 29)
  point P24 (-17.5, 29)
  point P25 (-12.5, 29)
  point P26 (-7.5, 29)
  point P27 (-2.5, 29)
  point P28 (2.5, 29)
  point P29 (7.5, 29)
  point P30 (12.5, 29)
  point P31 (17.5, 29)
  point P32 (22.5, 29)
  point P33 (27.5, 29)
  point P34 (32.5, 29)
  point P35 (37.5, 29)
  point P36 (-37.5, 23.5)
  point P37 (-32.5, 23.5)
  point P38 (-27.5, 23.5)
  point P39 (-22.5, 23.5)
  point P40 (-17.5, 23.5)
  point P41 (-12.5, 23.5)
  point P42 (-7.5, 23.5)
  point P43 (-2.5, 23.5)
  point P44 (2.5, 23.5)
  point P45 (7.5, 23.5)
  point P46 (12.5, 23.5)
  point P47 (17.5, 23.5)
  point P48 (22.5, 23.5)
  point P49 (27.5, 23.5)
  point P50 (32.5, 23.5)
  point P51 (37.5, 23.5)
  point P52 (-37.5, 18)
  point P53 (-32.5, 18)
  point P54 (-27.5, 18)
  point P55 (-22.5, 18)
  point P56 (-17.5, 18)
  point P57 (-12.5, 18)
  point P58 (-7.5, 18)
  point P59 (-2.5, 18)
  point P60 (2.5, 18)
  point P61 (7.5, 18)
  point P62 (12.5, 18)
  point P63 (17.5, 18)
  point P64 (22.5, 18)
  point P65 (27.5, 18)
  point P66 (32.5, 18)
  point P67 (37.5, 18)
  point P68 (0, 20.75)
  point P69 (0, 20.75)
  point P70 (-37.5, 12.5)
  point P71 (-32.5, 12.5)
  point P72 (-27.5, 12.5)
  point P73 (-22.5, 12.5)
  point P74 (-17.5, 12.5)
  point P75 (-12.5, 12.5)
  point P76 (-7.5, 12.5)
  point P77 (-2.5, 12.5)
  point P78 (2.5, 12.5)
  point P79 (7.5, 12.5)
  point P80 (12.5, 12.5)
  point P81 (17.5, 12.5)
  point P82 (22.5, 12.5)
  point P83 (27.5, 12.5)
  point P84 (32.5, 12.5)
  point P85 (37.5, 12.5)
  point P86 (-37.5, 7)
  point P87 (-32.5, 7)
  point P88 (-27.5, 7)
  point P89 (-22.5, 7)
  point P90 (-17.5, 7)
  point P91 (-12.5, 7)
  point P92 (-7.5, 7)
  point P93 (-2.5, 7)
  point P94 (2.5, 7)
  point P95 (7.5, 7)
  point P96 (12.5, 7)
  point P97 (17.5, 7)
  point P98 (22.5, 7)
  point P99 (27.5, 7)
  point P100 (32.5, 7)
  point P101 (37.5, 7)
  point P102 (0, 20.75)
  point P103 (39.5, 7)
  point P104 (39.5, 20.75)
  point P105 (0, 4.6906)
  dimension "d3" = 3.5
  dimension "d7" = 10
  dimension "d8" = 40
  dimension "d10" = 4
  dimension "d11" = 13
  dimension "d12" = 60
  dimension "d17" = 3
  dimension "d22" = 44
  dimension "d26" = 4
  dimension "d33" = 5
  dimension "d36" = 5.5
  constraints: 1184 end point, 9 midpoint, 8 coincident, 8 point on circle, 7 centre point, 6 horizontal, 6 point on line, 6 symmetric about line, 4 parallel, 4 perpendicular, 4 tangent, 4 vertical alignment, 3 vertical, 2 horizontal alignment, 1 collinear, 1 equal radius, 1254 other
  measures "d7" diameter of A1
  measures "d8" distance of A2.centre point (-20, 47)
  measures "d10" radius of A4
  measures "d11" distance from line of point (-20, 47) L3
  measures "d12" angle of L0 L3
  measures "d17" distance of L5.end L6.end
  measures "d22" distance from line of point (-20, 47) L5
  measures "d26" distance between parallel lines of L14 L11
  measures "d33" distance of L12.end L15.start
  measures "d36" distance of L12.end L105.start
extrude "Extrusion1" add sketch "Sketch1" along normal mid plane 30 contours L8 L5 L6 L0 | A4 L3 A5 L1 A7 L4 A6 L0 L6 L5 L8
extrude "Extrusion2" add sketch "Sketch1" along normal mid plane 18 contours A0 | A2
extrude "Extrusion3" add sketch "Sketch1" along normal blind 27.5 contours L8 L5 L6 L0
sketch "Sketch2" plane through (-55.2184, 3, 15) normal (0, 1, 0) x (1, 0, 0)
  line L0 (0, -12.5) -> (35.2184, -12.5) projected
  arc A0 (20.1092, -12.5) -> (15.1092, -12.5) centre (17.6092, -8.1699) ccw
  line L1 (35.2184, 0) -> (110.4367, 0) construction
  line L2 (35.2184, 0) -> (35.2184, -12.5) construction
  point P0 (55.2184, 15)
  point P1 (17.6092, -12.5)
  point P2 (17.6092, -3.1699)
  dimension "d21" = 5
  dimension "d25" = 5
  constraints: 3 point on circle, 2 point on line, 1 centre point, 1 midpoint, 1 vertical alignment
  measures "d21" radius of A0
  measures "d25" distance of A0.end A0.start
extrude "Extrusion4" cut sketch "Sketch2" against normal through all
body "Solid1"
